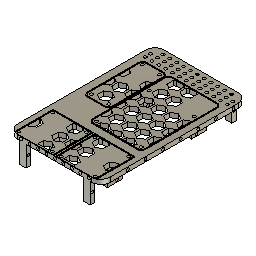
goose chassis v5 (Autodesk Fusion 360 design; units mm, degrees)
Autodesk Fusion 360 part; units mm, degrees
(part 1 of 2)
sketch "Sketch1" plane through (0, 0, 0) normal (0, 0, 1) x (1, 0, 0)
  line L0 (0, 0) -> (60, 0)
  line L1 (60, 0) -> (60, 100)
  line L2 (60, 100) -> (0, 100)
  line L3 (0, 100) -> (0, 0)
  line L4 (2, 92.9) -> (58, 92.9) construction
  line L5 (58, 92.9) -> (58, 7.1) construction
  line L6 (58, 7.1) -> (2, 7.1) construction
  line L7 (2, 7.1) -> (2, 92.9) construction
  line L8 (30, 92.9) -> (30, 7.1) construction
  line L9 (58, 50) -> (2, 50) construction
  line L10 (30, 100) -> (30, 0) construction
  line L11 (0, 50) -> (60, 50) construction
  line L12 (5.5, 89.5721) -> (54.5, 89.5721) construction
  line L13 (54.5, 89.5721) -> (54.5, 31.5721) construction
  line L14 (54.5, 31.5721) -> (5.5, 31.5721) construction
  line L15 (5.5, 31.5721) -> (5.5, 89.5721) construction
  line L16 (30, 89.5721) -> (30, 31.5721) construction
  circle A0 centre (5.5, 89.5721) radius 1.6
  circle A1 centre (54.5, 89.5721) radius 1.6
  circle A2 centre (54.5, 31.5721) radius 1.6
  circle A3 centre (5.5, 31.5721) radius 1.6
  line L17 (0, 100) -> (0, 140)
  line L18 (60, 100) -> (60, 140)
  line L19 (0, 140) -> (60, 140)
  dimension "d1" = 60
  dimension "d2" = 100
  dimension "d3" = 56
  dimension "d4" = 85.8
  dimension "d5" = 49
  dimension "d6" = 58
  dimension "d7" = 3.2
  dimension "d8" = 3.2
  dimension "d9" = 3.2
  dimension "d10" = 3.2
  dimension "d11" = 40
  dimension "d12" = 40
  constraint horizontal L0
  constraint vertical L1
  constraint horizontal L2
  constraint vertical L3
  constraint coincident L0.start L3.end
  constraint horizontal L4
  constraint vertical L5
  constraint horizontal L6
  constraint vertical L7
  constraint midpoint L4 L8.start
  constraint midpoint L6 L8.end
  constraint midpoint L5 L9.start
  constraint midpoint L7 L9.end
  constraint midpoint L2 L10.start
  constraint midpoint L0 L10.end
  constraint midpoint L3 L11.start
  constraint midpoint L1 L11.end
  constraint collinear L9 L11
  constraint collinear L8 L10
  constraint horizontal L12
  constraint vertical L13
  constraint horizontal L14
  constraint vertical L15
  constraint midpoint L12 L16.start
  constraint midpoint L14 L16.end
  constraint collinear L10 L16
  constraint coincident L12.start L15.end
  constraint coincident L12.end L13.start
  constraint coincident L13.end L14.start
  constraint coincident L14.end L15.start
  constraint perpendicular L2 L17
  constraint perpendicular L2 L18
  measures "d1" distance of L0.start L0.end
  measures "d2" distance of L0.start L2.end
  measures "d3" distance of L4.start L4.end
  measures "d4" distance of L4.start L6.end
  measures "d5" distance of L12.start L12.end
  measures "d6" distance of L12.start L14.end
  measures "d7" diameter of A0
  measures "d8" diameter of A1
  measures "d9" diameter of A2
  measures "d10" diameter of A3
  measures "d11" distance of L2.end L17.end
  measures "d12" distance of L1.end L18.end
extrude "Extrude1" add sketch "Sketch1" along normal blind 5 contours L0 L1 L2 L3 | L2 L17 L18 L19 | A0 | A1 | A2 | A3 makes body 1
sketch "Sketch2" plane through (0, 0, 0) normal (0, 0, 1) x (1, 0, 0)
  line L0 (0, 0) -> (19, 0) construction
  line L1 (19, 0) -> (19, 70) construction
  line L2 (19, 70) -> (0, 70) construction
  line L3 (0, 70) -> (0, 0) construction
  line L4 (9.5, 70) -> (9.5, 0) construction
  line L5 (19, 35) -> (0, 35) construction
  line L6 (19, 0) -> (12, 0)
  line L7 (12, 0) -> (12, 5)
  line L8 (12, 5) -> (19, 5)
  line L9 (19, 5) -> (19, 0)
  line L10 (19, 26) -> (29, 26)
  line L11 (29, 26) -> (29, 42)
  line L12 (29, 42) -> (19, 42)
  line L13 (19, 42) -> (19, 26)
  line L14 (0, 0) -> (60, 0) construction
  line L15 (60, 0) -> (60, 140) construction
  line L16 (60, 140) -> (0, 140) construction
  line L17 (0, 140) -> (0, 0) construction
  line L18 (30, 140) -> (30, 0) construction
  line L19 (60, 70) -> (0, 70) construction
  line L20 (41, 26) -> (31, 26)
  line L21 (31, 26) -> (31, 42)
  line L22 (41, 42) -> (41, 26)
  line L23 (31, 42) -> (41, 42)
  line L24 (41, 0) -> (48, 0)
  line L25 (48, 0) -> (48, 5)
  line L26 (41, 5) -> (41, 0)
  line L27 (48, 5) -> (41, 5)
  line L28 (41, 114) -> (31, 114)
  line L29 (31, 114) -> (31, 98)
  line L30 (41, 98) -> (41, 114)
  line L31 (31, 98) -> (41, 98)
  line L32 (19, 114) -> (29, 114)
  line L33 (29, 114) -> (29, 98)
  line L34 (19, 98) -> (19, 114)
  line L35 (29, 98) -> (19, 98)
  line L36 (19, 140) -> (12, 140)
  line L37 (12, 140) -> (12, 135)
  line L38 (19, 135) -> (19, 140)
  line L39 (12, 135) -> (19, 135)
  line L40 (41, 140) -> (48, 140)
  line L41 (48, 140) -> (48, 135)
  line L42 (41, 135) -> (41, 140)
  line L43 (48, 135) -> (41, 135)
  dimension "d15" = 19
  dimension "d16" = 70
  dimension "d17" = 7
  dimension "d18" = 5
  dimension "d19" = 12
  dimension "d20" = 10
  dimension "d21" = 16
  dimension "d22" = 42
  constraint horizontal L0
  constraint vertical L1
  constraint horizontal L2
  constraint vertical L3
  constraint coincident L0.start L3.end
  constraint midpoint L2 L4.start
  constraint midpoint L0 L4.end
  constraint midpoint L1 L5.start
  constraint midpoint L3 L5.end
  constraint horizontal L6
  constraint vertical L7
  constraint horizontal L8
  constraint vertical L9
  constraint coincident L0 L1.start
  constraint horizontal L10
  constraint vertical L11
  constraint horizontal L12
  constraint vertical L13
  constraint coincident L1 L10.start
  constraint horizontal L14
  constraint vertical L15
  constraint horizontal L16
  constraint vertical L17
  constraint midpoint L16 L18.start
  constraint midpoint L14 L18.end
  constraint midpoint L15 L19.start
  constraint perpendicular L3 L19
  constraint symmetric L0.end L18 L24.start
  constraint symmetric L6.end L18 L24.end
  constraint symmetric L7.end L18 L25.end
  constraint symmetric L8.end L18 L26.start
  constraint symmetric L10.start L18 L20.start
  constraint symmetric L10.end L18 L20.end
  constraint symmetric L11.end L18 L21.end
  constraint symmetric L12.end L18 L22.start
  constraint symmetric L0.end L19 L36.start
  constraint symmetric L6.end L19 L36.end
  constraint symmetric L7.end L19 L37.end
  constraint symmetric L8.end L19 L38.start
  constraint symmetric L10.start L19 L32.start
  constraint symmetric L10.end L19 L32.end
  constraint symmetric L11.end L19 L33.end
  constraint symmetric L12.end L19 L34.start
  constraint symmetric L19 L20.start L28.start
  constraint symmetric L19 L20.end L28.end
  constraint symmetric L19 L21.end L29.end
  constraint symmetric L19 L22.start L30.start
  constraint symmetric L19 L24.start L40.start
  constraint symmetric L19 L24.end L40.end
  constraint symmetric L19 L25.end L41.end
  constraint symmetric L19 L26.start L42.start
  measures "d15" distance of L0.start L0.end
  measures "d16" distance of L0.start L2.end
  measures "d17" distance of L0.end L6.end
  measures "d18" distance of L0.end L8.end
  measures "d19" distance of L3 L7
  measures "d20" distance of L10.start L10.end
  measures "d21" distance of L10.start L12.end
  measures "d22" distance of L12 L14
extrude "Extrude2" add sketch "Sketch2" against normal blind 22.5 bodies 1
sketch "Sketch3" plane through (12, 0, 0) normal (-1, 0, 0) x (0, -1, 0)
  line L0 (0, 0) -> (-5, 0)
  line L1 (-5, 0) -> (-5, -22.5)
  line L2 (-5, -22.5) -> (0, -22.5)
  line L3 (0, -22.5) -> (0, 0)
  line L4 (-2.5, 0) -> (-2.5, -11.5) construction
  circle A0 centre (-2.5, -11.5) radius 1.6
  circle A1 centre (-36.5, -2.5) radius 1.6
  circle A2 centre (-36.5, -20) radius 1.6
  line L5 (-140, 0) -> (0, 0)
  line L6 (-42, 0) -> (-42, -22.5)
  dimension "d25" = 11.5
  dimension "d26" = 3.2
  dimension "d27" = 3.2
  dimension "d28" = 3.2
  dimension "d29" = 2.5
  dimension "d30" = 5.5
  dimension "d31" = 20
  dimension "d32" = 5.5
  constraint midpoint L0 L4.start
  constraint perpendicular L0 L4
  constraint coincident L4.end A0.centre
  measures "d25" distance of L4.start L4.end
  measures "d26" diameter of A0
  measures "d27" diameter of A1
  measures "d28" diameter of A2
  measures "d29" distance of A1.centre L5
  measures "d30" distance of A1.centre L6
  measures "d31" distance of A2.centre L5
  measures "d32" distance of A2.centre L6
extrude "Extrude3" cut sketch "Sketch3" against normal blind 40 contours A0 | A1 | A2 bodies 1
ref_plane "WorkPlane1" through (30, 70, -8.75) normal (0, -1, 0) x (1, 0, 0)
mirror "Mirror1" about plane through (30, 70, -8.75) normal (0, -1, 0) of "Extrude3"
copy_body "Body->Comp1" bodies 1 removing the originals makes body 2 in component "chassis"
ref_plane "WorkPlane1" through (30, 80, -8.75) normal (0, -1, 0) x (1, 0, 0) in component "chassis"
split "Split1" by plane through (30, 80, -8.75) normal (0, -1, 0) bodies 2 makes body 3 at (20, 53.3333, 5) in component "chassis"
move_body "Move1" bodies 2 to x (1, 0, 0) y (0, 1, 0) z (0, 0, 1) at (0, 20, 0) in component "chassis"
loft "Loft1" add section 1 face at (20, 80, 1.6667) section 2 face at (20, 100, 1.6667) on bodies 2 3 bodies 2 3 in component "chassis"
ref_plane "WorkPlane2" through (30, 80, 2.5) normal (-1, 0, 0) x (0, -1, 0) in component "chassis"
split "Split2" by plane through (30, 80, 2.5) normal (-1, 0, 0) bodies 2 makes body 4 at (10, 106.6667, 5) in component "chassis"
move_body "Move2" bodies 2 to x (1, 0, 0) y (0, 1, 0) z (0, 0, 1) at (41, 0, 0) in component "chassis"
loft "Loft2" add section 1 face at (30, 53.3333, 3.3333) section 2 face at (71, 53.3333, 3.3333) on bodies 2 4 bodies 2 4 in component "chassis"
sketch "Sketch6" plane through (0, 0, 5) normal (0, 0, 1) x (-1, 0, 0)
  line L0 (-101, -160) -> (0, -160)
  line L1 (0, -160) -> (0, 0)
  line L2 (0, 0) -> (-101, 0)
  line L3 (-101, 0) -> (-101, -160)
  line L4 (-89.5, -55.4279) -> (-40.5, -55.4279) construction
  line L5 (-40.5, -55.4279) -> (-40.5, -113.4279) construction
  line L6 (-40.5, -113.4279) -> (-89.5, -113.4279) construction
  line L7 (-89.5, -113.4279) -> (-89.5, -55.4279) construction
  line L8 (-93, -52.1) -> (-37, -52.1) construction
  line L9 (-37, -52.1) -> (-37, -137.9) construction
  line L10 (-93, -137.9) -> (-93, -52.1) construction
  line L11 (-37, -137.9) -> (-93, -137.9) construction
  circle A0 centre (-40.5, -113.4279) radius 1.6
  circle A1 centre (-89.5, -113.4279) radius 1.6
  circle A2 centre (-40.5, -55.4279) radius 1.6
  circle A3 centre (-89.5, -55.4279) radius 1.6
  circle A4 centre (-54.9377, -39.4681) radius 1.6
  circle A5 centre (-54.9377, -2.6181) radius 1.6
  line L12 (0, -80) -> (-101, -80) construction
  line L13 (-31.1163, -133.9449) -> (-31.1163, -78.4449) construction
  line L14 (-31.1163, -78.4449) -> (-12.1163, -78.4449) construction
  line L15 (-12.1163, -78.4449) -> (-12.1163, -133.9449) construction
  line L16 (-12.1163, -133.9449) -> (-31.1163, -133.9449) construction
  line L17 (-34.8217, -137.6274) -> (-34.8217, -74.6274) construction
  line L18 (-34.8217, -74.6274) -> (-8.8217, -74.6274) construction
  line L19 (-8.8217, -74.6274) -> (-8.8217, -137.6274) construction
  line L20 (-8.8217, -137.6274) -> (-34.8217, -137.6274) construction
  circle A6 centre (-31.1163, -133.9449) radius 1.6
  circle A7 centre (-31.1163, -78.4449) radius 1.6
  circle A8 centre (-12.1163, -78.4449) radius 1.6
  circle A9 centre (-12.1163, -133.9449) radius 1.6
  circle A10 centre (-91.9377, -2.6181) radius 1.6
  circle A11 centre (-91.9377, -39.4681) radius 1.6
  line L21 (-101, 0) -> (0, 0) construction
  line L22 (0, 0) -> (0, -160) construction
  line L23 (0, -160) -> (-101, -160) construction
  line L24 (-101, -160) -> (-101, 0) construction
  line L25 (-50, 0) -> (-50.5, -160) construction
  circle A12 centre (-8.0795, -2.8802) radius 1.6
  circle A13 centre (-8.3098, -39.7295) radius 1.6
  circle A14 centre (-45.3091, -39.4982) radius 1.6
  circle A15 centre (-45.0788, -2.6489) radius 1.6
  dimension "d77" = 56
  dimension "d78" = 85.8
  dimension "d79" = 49
  dimension "d80" = 58
  dimension "d81" = 3.2
  dimension "d82" = 3.2
  dimension "d83" = 3.2
  dimension "d84" = 3.2
  dimension "d85" = 55.5
  dimension "d86" = 19
  dimension "d87" = 63
  dimension "d88" = 26
  dimension "d89" = 3.2
  dimension "d90" = 3.2
  dimension "d91" = 3.2
  dimension "d92" = 3.2
  constraint horizontal L8
  constraint vertical L9
  constraint horizontal L11
  constraint vertical L10
  constraint horizontal L4
  constraint vertical L5
  constraint horizontal L6
  constraint vertical L7
  constraint coincident L4.start L7.end
  constraint coincident L4.end L5.start
  constraint coincident L5.end L6.start
  constraint coincident L6.end L7.start
  constraint midpoint L1 L12.start
  constraint midpoint L3 L12.end
  constraint coincident L13.start L16.end
  constraint coincident L13.end L14.start
  constraint coincident L14.end L15.start
  constraint coincident L15.end L16.start
  constraint horizontal L21
  constraint vertical L22
  constraint horizontal L23
  constraint vertical L24
  constraint coincident L0.end L1.start
  constraint coincident L2.end L3.start
  constraint coincident L21 L25.start
  constraint midpoint L23 L25.end
  constraint symmetric A4 L25 A14
  constraint symmetric A5 L25 A15
  constraint symmetric A10 L25 A12
  constraint symmetric A11 L25 A13
  measures "d77" distance of L8.start L8.end
  measures "d78" distance of L8.start L10.start
  measures "d79" distance of L4.start L4.end
  measures "d80" distance of L6.end L4.start
  measures "d81" diameter of A3
  measures "d82" diameter of A2
  measures "d83" diameter of A0
  measures "d84" diameter of A1
  measures "d85" distance of L13.start L13.end
  measures "d86" distance of L13.start L15.end
  measures "d87" distance of L17.start L17.end
  measures "d88" distance of L17.start L19.end
  measures "d89" diameter of A6
  measures "d90" diameter of A7
  measures "d91" diameter of A8
  measures "d92" diameter of A9
extrude "Extrude1'" add sketch "Sketch6" against normal blind 5 contours A0 | A1 | A2 | A3 | A4 | A5 | A6 | A7 | A8 | A9 | A10 | A11 | A12 | A13 | A14 | A15 bodies 2 in component "chassis"
extrude "Extrude2'" cut sketch "Sketch6" against normal blind 5 contours A0 | A1 | A2 | A3 | A4 | A5 | A6 | A7 | A8 | A9 | A10 | A11 | A12 | A13 | A14 | A15 bodies 2 in component "chassis"
fillet "Fillet3" radius 10 4 edges at (101, 0, 2.5) (0, 0, 2.5) (0, 160, 2.5) (101, 160, 2.5) on bodies 2 in component "chassis"
sketch "Sketch7" plane through (0, 0, 5) normal (0, 0, 1) x (-1, 0, 0)
  circle A0 centre (-45.3091, -39.4982) radius 1.6
  circle A1 centre (-54.9377, -2.6181) radius 1.6
  circle A2 centre (-40.5, -55.4279) radius 1.6
  circle A3 centre (-89.5, -55.4279) radius 1.6
  circle A4 centre (-31.1163, -133.9449) radius 1.6
  circle A5 centre (-40.5, -113.4279) radius 1.6
  circle A6 centre (-8.3098, -39.7295) radius 1.6
  circle A7 centre (-91.9377, -39.4681) radius 1.6
  circle A8 centre (-45.0788, -2.6489) radius 1.6
  circle A9 centre (-12.1163, -78.4449) radius 1.6
  circle A10 centre (-31.1163, -78.4449) radius 1.6
  circle A11 centre (-54.9377, -39.4681) radius 1.6
  circle A12 centre (-12.1163, -133.9449) radius 1.6
  circle A13 centre (-89.5, -113.4279) radius 1.6
  circle A14 centre (-8.0795, -2.8802) radius 1.6
  circle A15 centre (-91.9377, -2.6181) radius 1.6
  arc A16 (-101, -150) -> (-91, -160) centre (-91, -150) ccw
  line L0 (-91, -160) -> (-10, -160)
  arc A17 (-10, -160) -> (0, -150) centre (-10, -150) ccw
  line L1 (0, -150) -> (0, -10)
  arc A18 (0, -10) -> (-10, 0) centre (-10, -10) ccw
  line L2 (-10, 0) -> (-91, 0)
  arc A19 (-91, 0) -> (-101, -10) centre (-91, -10) ccw
  line L3 (-101, -10) -> (-101, -150)
  line L4 (-91.9377, -2.6181) -> (-54.9377, -2.6181) construction
  line L5 (-54.9377, -2.6181) -> (-54.9377, -39.4681) construction
  line L6 (-54.9377, -39.4681) -> (-91.9377, -39.4681) construction
  line L7 (-91.9377, -39.4681) -> (-91.9377, -2.6181) construction
  line L8 (-94.4377, -41.9681) -> (-94.4377, -0.1181)
  line L9 (-94.4377, -0.1181) -> (-52.4377, -0.1181)
  line L10 (-52.4377, -0.1181) -> (-52.4377, -41.9681)
  line L11 (-52.4377, -41.9681) -> (-94.4377, -41.9681)
  line L12 (-41, -137.9) -> (-89, -137.9)
  line L13 (-93, -133.9) -> (-93, -56.1)
  line L14 (-89, -52.1) -> (-41, -52.1)
  line L15 (-37, -56.1) -> (-37, -133.9)
  line L16 (-12.8217, -137.6274) -> (-30.8217, -137.6274)
  line L17 (-34.8217, -133.6274) -> (-34.8217, -78.6274)
  line L18 (-30.8217, -74.6274) -> (-12.8217, -74.6274)
  line L19 (-8.8217, -78.6274) -> (-8.8217, -133.6274)
  arc A20 (-89, -52.1) -> (-93, -56.1) centre (-89, -56.1) ccw
  arc A21 (-37, -56.1) -> (-41, -52.1) centre (-41, -56.1) ccw
  arc A22 (-41, -137.9) -> (-37, -133.9) centre (-41, -133.9) ccw
  arc A23 (-93, -133.9) -> (-89, -137.9) centre (-89, -133.9) ccw
  arc A24 (-34.8217, -133.6274) -> (-30.8217, -137.6274) centre (-30.8217, -133.6274) ccw
  arc A25 (-12.8217, -137.6274) -> (-8.8217, -133.6274) centre (-12.8217, -133.6274) ccw
  arc A26 (-8.8217, -78.6274) -> (-12.8217, -74.6274) centre (-12.8217, -78.6274) ccw
  arc A27 (-30.8217, -74.6274) -> (-34.8217, -78.6274) centre (-30.8217, -78.6274) ccw
  line L20 (-50.5, 0) -> (-50.5, -160) construction
  line L21 (-6.5623, -41.9681) -> (-6.5623, -0.1181)
  line L22 (-6.5623, -0.1181) -> (-48.5623, -0.1181)
  line L23 (-48.5623, -0.1181) -> (-48.5623, -41.9681)
  line L24 (-48.5623, -41.9681) -> (-6.5623, -41.9681)
  line L25 (-95.4377, 0.8819) -> (-51.4377, 0.8819)
  line L26 (-51.4377, 0.8819) -> (-51.4377, -42.9681)
  line L27 (-51.4377, -42.9681) -> (-95.4377, -42.9681)
  line L28 (-95.4377, -42.9681) -> (-95.4377, 0.8819)
  line L29 (-5.5623, 0.8819) -> (-49.5623, 0.8819)
  line L30 (-49.5623, 0.8819) -> (-49.5623, -42.9681)
  line L31 (-49.5623, -42.9681) -> (-5.5623, -42.9681)
  line L32 (-5.5623, -42.9681) -> (-5.5623, 0.8819)
  arc A28 (-36, -56.1) -> (-41, -51.1) centre (-41, -56.1) ccw
  line L33 (-89, -51.1) -> (-41, -51.1)
  arc A29 (-89, -51.1) -> (-94, -56.1) centre (-89, -56.1) ccw
  line L34 (-94, -133.9) -> (-94, -56.1)
  arc A30 (-94, -133.9) -> (-89, -138.9) centre (-89, -133.9) ccw
  line L35 (-41, -138.9) -> (-89, -138.9)
  arc A31 (-41, -138.9) -> (-36, -133.9) centre (-41, -133.9) ccw
  line L36 (-36, -56.1) -> (-36, -133.9)
  arc A32 (-7.8217, -78.6274) -> (-12.8217, -73.6274) centre (-12.8217, -78.6274) ccw
  line L37 (-30.8217, -73.6274) -> (-12.8217, -73.6274)
  arc A33 (-30.8217, -73.6274) -> (-35.8217, -78.6274) centre (-30.8217, -78.6274) ccw
  line L38 (-35.8217, -133.6274) -> (-35.8217, -78.6274)
  arc A34 (-35.8217, -133.6274) -> (-30.8217, -138.6274) centre (-30.8217, -133.6274) ccw
  line L39 (-12.8217, -138.6274) -> (-30.8217, -138.6274)
  arc A35 (-12.8217, -138.6274) -> (-7.8217, -133.6274) centre (-12.8217, -133.6274) ccw
  line L40 (-7.8217, -78.6274) -> (-7.8217, -133.6274)
  point P0 (-93.0412, -137.3397)
  point P1 (-93.0412, -51.5397)
  point P2 (-37.0412, -51.5397)
  point P3 (-34.8217, -127.6274)
  point P4 (-8.8217, -127.6274)
  point P5 (-93, -137.9)
  point P6 (-93, -52.1)
  point P7 (-37, -52.1)
  point P8 (-34.8217, -137.6274)
  point P9 (-34.8217, -74.6274)
  point P10 (-8.8217, -137.6274)
  dimension "d112" = -2.5
  dimension "d113" = 56
  dimension "d114" = 85.8
  dimension "d115" = 63
  dimension "d116" = 26
  dimension "d117" = 4
  dimension "d118" = -1
  dimension "d119" = 1
  dimension "d120" = -1
  dimension "d121" = -1
  constraint horizontal L4
  constraint vertical L5
  constraint horizontal L6
  constraint vertical L7
  constraint coincident A11.centre L5.end
  constraint coincident A15.centre L4.start
  constraint horizontal L14
  constraint vertical L15
  constraint horizontal L12
  constraint vertical L13
  constraint coincident P6 L13
  constraint coincident P6 L14
  constraint tangent L13 A20
  constraint tangent L14 A20
  constraint coincident P7 L14
  constraint coincident P7 L15
  constraint tangent L14 A21
  constraint tangent L15 A21
  constraint equal A20 A21
  constraint tangent L12 A22
  constraint tangent L15 A22
  constraint equal A20 A22
  constraint coincident P5 L12
  constraint coincident P5 L13
  constraint tangent L12 A23
  constraint tangent L13 A23
  constraint equal A20 A23
  constraint coincident P8 L16
  constraint coincident P8 L17
  constraint tangent L16 A24
  constraint tangent L17 A24
  constraint equal A20 A24
  constraint coincident P10 L16
  constraint coincident P10 L19
  constraint tangent L16 A25
  constraint tangent L19 A25
  constraint equal A20 A25
  constraint tangent L18 A26
  constraint tangent L19 A26
  constraint equal A20 A26
  constraint coincident P9 L17
  constraint coincident P9 L18
  constraint tangent L17 A27
  constraint tangent L18 A27
  constraint equal A20 A27
  constraint midpoint L2 L20.start
  constraint midpoint L0 L20.end
  constraint symmetric L8.start L20 L21.start
  constraint symmetric L8.end L20 L21.end
  constraint symmetric L9.end L20 L22.end
  constraint symmetric L10.end L20 L23.end
  measures "d113" distance of P6 P7
  measures "d114" distance of P5 P6
  measures "d115" distance of P8 P9
  measures "d116" distance of P8 P10
  measures "d117" radius of A20
extrude "Extrude3'" cut sketch "Sketch7" against normal blind 0.5 contours A14 A18 L2 L21 L22 L23 L24 L30 L31 L32 | L2 A19 L8 L9 L10 L11 L26 L27 L28 | A28 L33 A29 L34 A30 L35 A31 L36 | A32 L37 A33 L38 A34 L39 A35 L40 bodies 2 in component "chassis"
sketch "Sketch8" plane through (0, 0, 5) normal (0, 0, 1) x (-1, 0, 0)
  line L0 (-95.4377, -42.9681) -> (-95.4377, -1.0386)
  arc A0 (-95.4377, -1.0386) -> (-101, -10) centre (-91, -10) ccw
  line L1 (-101, -10) -> (-101, -150)
  arc A1 (-101, -150) -> (-91, -160) centre (-91, -150) ccw
  line L2 (-91, -160) -> (-10, -160)
  arc A2 (-10, -160) -> (0, -150) centre (-10, -150) ccw
  line L3 (0, -150) -> (0, -10)
  arc A3 (0, -10) -> (-5.5623, -1.0386) centre (-10, -10) ccw
  line L4 (-5.5623, -1.0386) -> (-5.5623, -42.9681)
  line L5 (-5.5623, -42.9681) -> (-49.5623, -42.9681)
  line L6 (-49.5623, -42.9681) -> (-49.5623, 0)
  line L7 (-49.5623, 0) -> (-51.4377, 0)
  line L8 (-51.4377, 0) -> (-51.4377, -42.9681)
  line L9 (-51.4377, -42.9681) -> (-95.4377, -42.9681)
  line L10 (-94, -133.9) -> (-94, -56.1)
  arc A4 (-89, -51.1) -> (-94, -56.1) centre (-89, -56.1) ccw
  line L11 (-89, -51.1) -> (-41, -51.1)
  arc A5 (-36, -56.1) -> (-41, -51.1) centre (-41, -56.1) ccw
  line L12 (-36, -56.1) -> (-36, -133.9)
  arc A6 (-41, -138.9) -> (-36, -133.9) centre (-41, -133.9) ccw
  line L13 (-41, -138.9) -> (-89, -138.9)
  arc A7 (-94, -133.9) -> (-89, -138.9) centre (-89, -133.9) ccw
  line L14 (-35.8217, -133.6274) -> (-35.8217, -78.6274)
  arc A8 (-30.8217, -73.6274) -> (-35.8217, -78.6274) centre (-30.8217, -78.6274) ccw
  line L15 (-30.8217, -73.6274) -> (-12.8217, -73.6274)
  arc A9 (-7.8217, -78.6274) -> (-12.8217, -73.6274) centre (-12.8217, -78.6274) ccw
  line L16 (-7.8217, -78.6274) -> (-7.8217, -133.6274)
  arc A10 (-12.8217, -138.6274) -> (-7.8217, -133.6274) centre (-12.8217, -133.6274) ccw
  line L17 (-12.8217, -138.6274) -> (-30.8217, -138.6274)
  arc A11 (-35.8217, -133.6274) -> (-30.8217, -138.6274) centre (-30.8217, -133.6274) ccw
  line L18 (-65, -51.1) -> (-65, -138.9) construction
  line L19 (-36, -95) -> (-94, -95) construction
  line L20 (-21.8217, -73.6274) -> (-21.8217, -138.6274) construction
  line L21 (-35.8217, -106.1274) -> (-7.8217, -106.1274) construction
  line L22 (-95.4377, -22.0034) -> (-51.4377, -21.4841) construction
  line L23 (-73.4377, -42.9681) -> (-73.4377, 0) construction
  line L24 (-94.007, -10.6431) -> (-92.5355, -11.4927)
  line L25 (-92.5355, -11.4927) -> (-86.5355, -8.0286)
  line L26 (-86.5355, -8.0286) -> (-86.5355, -2.0505)
  line L27 (-84.3689, -2.0505) -> (-84.3689, -8.0286)
  line L28 (-84.3689, -8.0286) -> (-78.3689, -11.4927)
  line L29 (-78.3689, -11.4927) -> (-72.3689, -8.0286)
  line L30 (-72.3689, -8.0286) -> (-72.3689, -2.0505)
  line L31 (-70.2022, -2.0505) -> (-70.2022, -8.0286)
  line L32 (-70.2022, -8.0286) -> (-64.2022, -11.4927)
  line L33 (-64.2022, -11.4927) -> (-58.2022, -8.0286)
  line L34 (-58.2022, -8.0286) -> (-58.2022, -2.0505)
  line L35 (-41.8689, -2.0505) -> (-41.8689, -8.0286)
  line L36 (-41.8689, -8.0286) -> (-35.8689, -11.4927)
  line L37 (-35.8689, -11.4927) -> (-29.8689, -8.0286)
  line L38 (-29.8689, -8.0286) -> (-29.8689, -2.0505)
  line L39 (-27.7022, -2.0505) -> (-27.7022, -8.0286)
  line L40 (-27.7022, -8.0286) -> (-21.7022, -11.4927)
  line L41 (-21.7022, -11.4927) -> (-15.7022, -8.0286)
  line L42 (-15.7022, -8.0286) -> (-15.7022, -2.0505)
  line L43 (-13.5355, -2.0505) -> (-13.5355, -8.0286)
  line L44 (-13.5355, -8.0286) -> (-7.5355, -11.4927)
  line L45 (-7.5355, -11.4927) -> (-7, -11.1835)
  line L46 (-94.007, -26.6431) -> (-92.5355, -27.4927)
  line L47 (-92.5355, -27.4927) -> (-86.5355, -24.0286)
  line L48 (-86.5355, -24.0286) -> (-86.5355, -17.1004)
  line L49 (-92.5355, -13.6363) -> (-94.007, -14.4858)
  line L50 (-86.5355, -17.1004) -> (-92.5355, -13.6363)
  line L51 (-84.3689, -17.1004) -> (-84.3689, -24.0286)
  line L52 (-84.3689, -24.0286) -> (-78.3689, -27.4927)
  line L53 (-78.3689, -27.4927) -> (-72.3689, -24.0286)
  line L54 (-72.3689, -24.0286) -> (-72.3689, -17.1004)
  line L55 (-78.3689, -13.6363) -> (-84.3689, -17.1004)
  line L56 (-72.3689, -17.1004) -> (-78.3689, -13.6363)
  line L57 (-70.2022, -17.1004) -> (-70.2022, -24.0286)
  line L58 (-70.2022, -24.0286) -> (-64.2022, -27.4927)
  line L59 (-64.2022, -27.4927) -> (-58.2022, -24.0286)
  line L60 (-58.2022, -24.0286) -> (-58.2022, -17.1004)
  line L61 (-64.2022, -13.6363) -> (-70.2022, -17.1004)
  line L62 (-58.2022, -17.1004) -> (-64.2022, -13.6363)
  line L63 (-56.0355, -17.1004) -> (-56.0355, -24.0286)
  line L64 (-44.0355, -24.0286) -> (-44.0355, -17.1004)
  line L65 (-44.0355, -17.1004) -> (-47.9856, -14.8198)
  line L66 (-41.8689, -17.1004) -> (-41.8689, -24.0286)
  line L67 (-41.8689, -24.0286) -> (-35.8689, -27.4927)
  line L68 (-35.8689, -27.4927) -> (-29.8689, -24.0286)
  line L69 (-29.8689, -24.0286) -> (-29.8689, -17.1004)
  line L70 (-35.8689, -13.6363) -> (-41.8689, -17.1004)
  line L71 (-29.8689, -17.1004) -> (-35.8689, -13.6363)
  line L72 (-27.7022, -17.1004) -> (-27.7022, -24.0286)
  line L73 (-27.7022, -24.0286) -> (-21.7022, -27.4927)
  line L74 (-21.7022, -27.4927) -> (-15.7022, -24.0286)
  line L75 (-15.7022, -24.0286) -> (-15.7022, -17.1004)
  line L76 (-21.7022, -13.6363) -> (-27.7022, -17.1004)
  line L77 (-15.7022, -17.1004) -> (-21.7022, -13.6363)
  line L78 (-13.5355, -17.1004) -> (-13.5355, -24.0286)
  line L79 (-13.5355, -24.0286) -> (-7.5355, -27.4927)
  line L80 (-7.5355, -13.6363) -> (-13.5355, -17.1004)
  line L81 (-7, -13.9455) -> (-7.5355, -13.6363)
  line L82 (-84.3689, -33.1004) -> (-84.3689, -40.0286)
  line L83 (-72.3689, -40.0286) -> (-72.3689, -33.1004)
  line L84 (-78.3689, -29.6363) -> (-84.3689, -33.1004)
  line L85 (-72.3689, -33.1004) -> (-78.3689, -29.6363)
  line L86 (-70.2022, -33.1004) -> (-70.2022, -40.0286)
  line L87 (-60.7508, -41.5) -> (-58.2022, -40.0286)
  line L88 (-58.2022, -40.0286) -> (-58.2022, -33.1004)
  line L89 (-64.2022, -29.6363) -> (-70.2022, -33.1004)
  line L90 (-58.2022, -33.1004) -> (-64.2022, -29.6363)
  line L91 (-41.8689, -33.1004) -> (-41.8689, -40.0286)
  line L92 (-29.8689, -40.0286) -> (-29.8689, -33.1004)
  line L93 (-35.8689, -29.6363) -> (-41.8689, -33.1004)
  line L94 (-29.8689, -33.1004) -> (-35.8689, -29.6363)
  line L95 (-27.7022, -33.1004) -> (-27.7022, -40.0286)
  line L96 (-15.7022, -40.0286) -> (-15.7022, -33.1004)
  line L97 (-21.7022, -29.6363) -> (-27.7022, -33.1004)
  line L98 (-15.7022, -33.1004) -> (-21.7022, -29.6363)
  line L99 (-84.3689, -52.5645) -> (-84.3689, -56.0286)
  line L100 (-84.3689, -56.0286) -> (-78.3689, -59.4927)
  line L101 (-78.3689, -59.4927) -> (-72.3689, -56.0286)
  line L102 (-72.3689, -56.0286) -> (-72.3689, -52.5645)
  line L103 (-70.2022, -52.5645) -> (-70.2022, -56.0286)
  line L104 (-70.2022, -56.0286) -> (-64.2022, -59.4927)
  line L105 (-64.2022, -59.4927) -> (-58.2022, -56.0286)
  line L106 (-58.2022, -56.0286) -> (-58.2022, -52.5645)
  line L107 (-56.0355, -52.5645) -> (-56.0355, -56.0286)
  line L108 (-56.0355, -56.0286) -> (-50.0355, -59.4927)
  line L109 (-50.0355, -59.4927) -> (-44.0355, -56.0286)
  line L110 (-44.0355, -56.0286) -> (-44.0355, -52.5645)
  line L111 (-92.5355, -75.4927) -> (-86.5355, -72.0286)
  line L112 (-86.5355, -72.0286) -> (-86.5355, -65.1004)
  line L113 (-86.5355, -65.1004) -> (-92.5355, -61.6363)
  line L114 (-84.3689, -65.1004) -> (-84.3689, -72.0286)
  line L115 (-84.3689, -72.0286) -> (-78.3689, -75.4927)
  line L116 (-78.3689, -75.4927) -> (-72.3689, -72.0286)
  line L117 (-72.3689, -72.0286) -> (-72.3689, -65.1004)
  line L118 (-78.3689, -61.6363) -> (-84.3689, -65.1004)
  line L119 (-72.3689, -65.1004) -> (-78.3689, -61.6363)
  line L120 (-70.2022, -65.1004) -> (-70.2022, -72.0286)
  line L121 (-70.2022, -72.0286) -> (-64.2022, -75.4927)
  line L122 (-64.2022, -75.4927) -> (-58.2022, -72.0286)
  line L123 (-58.2022, -72.0286) -> (-58.2022, -65.1004)
  line L124 (-64.2022, -61.6363) -> (-70.2022, -65.1004)
  line L125 (-58.2022, -65.1004) -> (-64.2022, -61.6363)
  line L126 (-56.0355, -65.1004) -> (-56.0355, -72.0286)
  line L127 (-56.0355, -72.0286) -> (-50.0355, -75.4927)
  line L128 (-50.0355, -75.4927) -> (-44.0355, -72.0286)
  line L129 (-44.0355, -72.0286) -> (-44.0355, -65.1004)
  line L130 (-50.0355, -61.6363) -> (-56.0355, -65.1004)
  line L131 (-44.0355, -65.1004) -> (-50.0355, -61.6363)
  line L132 (-41.8689, -65.1004) -> (-41.8689, -72.0286)
  line L133 (-92.5355, -91.4927) -> (-86.5355, -88.0286)
  line L134 (-86.5355, -88.0286) -> (-86.5355, -81.1004)
  line L135 (-86.5355, -81.1004) -> (-92.5355, -77.6363)
  line L136 (-84.3689, -81.1004) -> (-84.3689, -88.0286)
  line L137 (-84.3689, -88.0286) -> (-78.3689, -91.4927)
  line L138 (-78.3689, -91.4927) -> (-72.3689, -88.0286)
  line L139 (-72.3689, -88.0286) -> (-72.3689, -81.1004)
  line L140 (-78.3689, -77.6363) -> (-84.3689, -81.1004)
  line L141 (-72.3689, -81.1004) -> (-78.3689, -77.6363)
  line L142 (-70.2022, -81.1004) -> (-70.2022, -88.0286)
  line L143 (-70.2022, -88.0286) -> (-64.2022, -91.4927)
  line L144 (-64.2022, -91.4927) -> (-58.2022, -88.0286)
  line L145 (-58.2022, -88.0286) -> (-58.2022, -81.1004)
  line L146 (-64.2022, -77.6363) -> (-70.2022, -81.1004)
  line L147 (-58.2022, -81.1004) -> (-64.2022, -77.6363)
  line L148 (-56.0355, -81.1004) -> (-56.0355, -88.0286)
  line L149 (-56.0355, -88.0286) -> (-50.0355, -91.4927)
  line L150 (-50.0355, -91.4927) -> (-44.0355, -88.0286)
  line L151 (-44.0355, -88.0286) -> (-44.0355, -81.1004)
  line L152 (-50.0355, -77.6363) -> (-56.0355, -81.1004)
  line L153 (-44.0355, -81.1004) -> (-50.0355, -77.6363)
  line L154 (-41.8689, -81.1004) -> (-41.8689, -88.0286)
  line L155 (-27.7022, -81.1004) -> (-27.7022, -88.0286)
  line L156 (-27.7022, -88.0286) -> (-21.7022, -91.4927)
  line L157 (-21.7022, -91.4927) -> (-15.7022, -88.0286)
  line L158 (-15.7022, -88.0286) -> (-15.7022, -81.1004)
  line L159 (-21.7022, -77.6363) -> (-27.7022, -81.1004)
  line L160 (-15.7022, -81.1004) -> (-21.7022, -77.6363)
  line L161 (-92.5355, -107.4927) -> (-86.5355, -104.0286)
  line L162 (-86.5355, -104.0286) -> (-86.5355, -97.1004)
  line L163 (-86.5355, -97.1004) -> (-92.5355, -93.6363)
  line L164 (-84.3689, -97.1004) -> (-84.3689, -104.0286)
  line L165 (-84.3689, -104.0286) -> (-78.3689, -107.4927)
  line L166 (-78.3689, -107.4927) -> (-72.3689, -104.0286)
  line L167 (-72.3689, -104.0286) -> (-72.3689, -97.1004)
  line L168 (-78.3689, -93.6363) -> (-84.3689, -97.1004)
  line L169 (-72.3689, -97.1004) -> (-78.3689, -93.6363)
  line L170 (-70.2022, -97.1004) -> (-70.2022, -104.0286)
  line L171 (-70.2022, -104.0286) -> (-64.2022, -107.4927)
  line L172 (-64.2022, -107.4927) -> (-58.2022, -104.0286)
  line L173 (-58.2022, -104.0286) -> (-58.2022, -97.1004)
  line L174 (-64.2022, -93.6363) -> (-70.2022, -97.1004)
  line L175 (-58.2022, -97.1004) -> (-64.2022, -93.6363)
  line L176 (-56.0355, -97.1004) -> (-56.0355, -104.0286)
  line L177 (-56.0355, -104.0286) -> (-50.0355, -107.4927)
  line L178 (-50.0355, -107.4927) -> (-44.0355, -104.0286)
  line L179 (-44.0355, -104.0286) -> (-44.0355, -97.1004)
  line L180 (-50.0355, -93.6363) -> (-56.0355, -97.1004)
  line L181 (-44.0355, -97.1004) -> (-50.0355, -93.6363)
  line L182 (-41.8689, -97.1004) -> (-41.8689, -104.0286)
  line L183 (-34.3572, -106.6199) -> (-29.8689, -104.0286)
  line L184 (-29.8689, -104.0286) -> (-29.8689, -97.1004)
  line L185 (-29.8689, -97.1004) -> (-34.3572, -94.509)
  line L186 (-27.7022, -97.1004) -> (-27.7022, -104.0286)
  line L187 (-27.7022, -104.0286) -> (-21.7022, -107.4927)
  line L188 (-21.7022, -107.4927) -> (-15.7022, -104.0286)
  line L189 (-15.7022, -104.0286) -> (-15.7022, -97.1004)
  line L190 (-21.7022, -93.6363) -> (-27.7022, -97.1004)
  line L191 (-15.7022, -97.1004) -> (-21.7022, -93.6363)
  line L192 (-13.5355, -97.1004) -> (-13.5355, -104.0286)
  line L193 (-9.2861, -94.647) -> (-13.5355, -97.1004)
  line L194 (-92.5355, -123.4927) -> (-86.5355, -120.0286)
  line L195 (-86.5355, -120.0286) -> (-86.5355, -113.1004)
  line L196 (-86.5355, -113.1004) -> (-92.5355, -109.6363)
  line L197 (-84.3689, -113.1004) -> (-84.3689, -120.0286)
  line L198 (-84.3689, -120.0286) -> (-78.3689, -123.4927)
  line L199 (-78.3689, -123.4927) -> (-72.3689, -120.0286)
  line L200 (-72.3689, -120.0286) -> (-72.3689, -113.1004)
  line L201 (-78.3689, -109.6363) -> (-84.3689, -113.1004)
  line L202 (-72.3689, -113.1004) -> (-78.3689, -109.6363)
  line L203 (-70.2022, -113.1004) -> (-70.2022, -120.0286)
  line L204 (-70.2022, -120.0286) -> (-64.2022, -123.4927)
  line L205 (-64.2022, -123.4927) -> (-58.2022, -120.0286)
  line L206 (-58.2022, -120.0286) -> (-58.2022, -113.1004)
  line L207 (-64.2022, -109.6363) -> (-70.2022, -113.1004)
  line L208 (-58.2022, -113.1004) -> (-64.2022, -109.6363)
  line L209 (-56.0355, -113.1004) -> (-56.0355, -120.0286)
  line L210 (-56.0355, -120.0286) -> (-50.0355, -123.4927)
  line L211 (-50.0355, -123.4927) -> (-44.0355, -120.0286)
  line L212 (-44.0355, -120.0286) -> (-44.0355, -113.1004)
  line L213 (-50.0355, -109.6363) -> (-56.0355, -113.1004)
  line L214 (-44.0355, -113.1004) -> (-50.0355, -109.6363)
  line L215 (-41.8689, -113.1004) -> (-41.8689, -120.0286)
  line L216 (-29.8689, -120.0286) -> (-29.8689, -113.1004)
  line L217 (-29.8689, -113.1004) -> (-34.3572, -110.509)
  line L218 (-27.7022, -113.1004) -> (-27.7022, -120.0286)
  line L219 (-27.7022, -120.0286) -> (-21.7022, -123.4927)
  line L220 (-21.7022, -123.4927) -> (-15.7022, -120.0286)
  line L221 (-15.7022, -120.0286) -> (-15.7022, -113.1004)
  line L222 (-21.7022, -109.6363) -> (-27.7022, -113.1004)
  line L223 (-15.7022, -113.1004) -> (-21.7022, -109.6363)
  line L224 (-13.5355, -113.1004) -> (-13.5355, -120.0286)
  line L225 (-13.5355, -120.0286) -> (-9.2861, -122.482)
  line L226 (-9.2861, -110.647) -> (-13.5355, -113.1004)
  line L227 (-84.3689, -129.1004) -> (-84.3689, -136.0286)
  line L228 (-72.3689, -136.0286) -> (-72.3689, -129.1004)
  line L229 (-78.3689, -125.6363) -> (-84.3689, -129.1004)
  line L230 (-72.3689, -129.1004) -> (-78.3689, -125.6363)
  line L231 (-70.2022, -129.1004) -> (-70.2022, -136.0286)
  line L232 (-60.6391, -137.4355) -> (-58.2022, -136.0286)
  line L233 (-58.2022, -136.0286) -> (-58.2022, -129.1004)
  line L234 (-64.2022, -125.6363) -> (-70.2022, -129.1004)
  line L235 (-58.2022, -129.1004) -> (-64.2022, -125.6363)
  line L236 (-56.0355, -129.1004) -> (-56.0355, -136.0286)
  line L237 (-46.4725, -137.4355) -> (-44.0355, -136.0286)
  line L238 (-44.0355, -136.0286) -> (-44.0355, -129.1004)
  line L239 (-50.0355, -125.6363) -> (-56.0355, -129.1004)
  line L240 (-44.0355, -129.1004) -> (-50.0355, -125.6363)
  line L241 (-27.7022, -129.1004) -> (-27.7022, -136.0286)
  line L242 (-27.7022, -136.0286) -> (-25.7374, -137.163)
  line L243 (-17.667, -137.163) -> (-15.7022, -136.0286)
  line L244 (-15.7022, -136.0286) -> (-15.7022, -129.1004)
  line L245 (-21.7022, -125.6363) -> (-27.7022, -129.1004)
  line L246 (-15.7022, -129.1004) -> (-21.7022, -125.6363)
  line L247 (-37.5281, -62.5942) -> (-41.8689, -65.1004)
  line L248 (-41.8689, -72.0286) -> (-37.6035, -74.4912)
  line L249 (-84.3689, -136.0286) -> (-81.9319, -137.4355)
  line L250 (-74.8058, -137.4355) -> (-72.3689, -136.0286)
  line L251 (-70.2022, -136.0286) -> (-67.7653, -137.4355)
  line L252 (-56.0355, -136.0286) -> (-53.5986, -137.4355)
  line L253 (-50.5, 0) -> (-50.5, -138.9) construction
  line L254 (-50.5, -139.2245) -> (-50.5, -160) construction
  line L255 (-41.8689, -120.0286) -> (-37.9069, -122.316)
  line L256 (-36, -123.417) -> (-35.8689, -123.4927)
  line L257 (-37.8336, -110.7706) -> (-41.8689, -113.1004)
  line L258 (-41.8689, -104.0286) -> (-37.8058, -106.3744)
  line L259 (-37.7318, -94.7118) -> (-41.8689, -97.1004)
  line L260 (-41.8689, -88.0286) -> (-37.7046, -90.4328)
  line L261 (-37.6299, -78.653) -> (-41.8689, -81.1004)
  line L262 (-84.3689, -52.5645) -> (-72.3689, -52.5645)
  line L263 (-70.2022, -52.5645) -> (-58.2022, -52.5645)
  line L264 (-56.0355, -52.5645) -> (-44.0355, -52.5645)
  line L265 (-92.5355, -75.4927) -> (-92.5355, -61.6363)
  line L266 (-92.5355, -91.4927) -> (-92.5355, -77.6363)
  line L267 (-37.5281, -62.5942) -> (-37.6035, -74.4912)
  line L268 (-37.6299, -78.653) -> (-37.7046, -90.4328)
  line L269 (-37.7318, -94.7118) -> (-37.8058, -106.3744)
  line L270 (-37.8336, -110.7706) -> (-37.9069, -122.316)
  line L271 (-53.5986, -137.4355) -> (-46.4725, -137.4355)
  line L272 (-67.7653, -137.4355) -> (-60.6391, -137.4355)
  line L273 (-81.9319, -137.4355) -> (-74.8058, -137.4355)
  line L274 (-92.5355, -123.4927) -> (-92.5355, -109.6363)
  line L275 (-92.5355, -107.4927) -> (-92.5355, -93.6363)
  line L276 (-35.7372, -77.7123) -> (-35.8689, -77.6363)
  line L277 (-13.5355, -104.0286) -> (-9.2861, -106.482)
  line L278 (-7.8217, -107.3275) -> (-7.5355, -107.4927)
  line L279 (-9.2861, -94.647) -> (-9.2861, -106.482)
  line L280 (-9.2861, -110.647) -> (-9.2861, -122.482)
  line L281 (-34.3572, -106.6199) -> (-34.3572, -94.509)
  line L282 (-17.667, -137.163) -> (-25.7374, -137.163)
  line L283 (-34.3572, -122.6199) -> (-34.3572, -110.509)
  line L284 (-35.8689, -123.4927) -> (-35.8217, -123.4654)
  line L285 (-34.3572, -122.6199) -> (-29.8689, -120.0286)
  line L286 (-35.8217, -125.6635) -> (-35.8689, -125.6363)
  line L287 (-84.3689, -40.0286) -> (-81.8203, -41.5)
  line L288 (-74.9175, -41.5) -> (-72.3689, -40.0286)
  line L289 (-70.2022, -40.0286) -> (-67.6536, -41.5)
  line L290 (-56.0355, -24.0286) -> (-53, -25.7811)
  line L291 (-47.9856, -26.3092) -> (-44.0355, -24.0286)
  line L292 (-60.7508, -41.5) -> (-67.6536, -41.5)
  line L293 (-74.9175, -41.5) -> (-81.8203, -41.5)
  line L294 (-94.007, -26.6431) -> (-94.007, -14.4858)
  line L295 (-53, -15.3478) -> (-53, -25.7811)
  line L296 (-53, -15.3478) -> (-56.0355, -17.1004)
  line L297 (-47.9856, -26.3092) -> (-47.9856, -14.8198)
  line L298 (-32.4175, -41.5) -> (-39.3203, -41.5)
  line L299 (-32.4175, -41.5) -> (-29.8689, -40.0286)
  line L300 (-41.8689, -40.0286) -> (-39.3203, -41.5)
  line L301 (-27.7022, -40.0286) -> (-25.1536, -41.5)
  line L302 (-18.2508, -41.5) -> (-15.7022, -40.0286)
  line L303 (-18.2508, -41.5) -> (-25.1536, -41.5)
  line L304 (-7.5355, -27.4927) -> (-7, -27.1835)
  line L305 (-7, -13.9455) -> (-7, -27.1835)
  line L306 (-89.0676, -2.0505) -> (-89.0676, -5.5)
  line L307 (-89.0676, -5.5) -> (-94, -5.5)
  line L308 (-11, -2.0505) -> (-11, -5)
  line L309 (-11, -5) -> (-11, -6)
  line L310 (-11, -6) -> (-7, -6)
  line L311 (-94.007, -10.6431) -> (-94, -5.5)
  line L312 (-89.0676, -2.0505) -> (-86.5355, -2.0505)
  line L313 (-84.3689, -2.0505) -> (-72.3689, -2.0505)
  line L314 (-70.2022, -2.0505) -> (-58.2022, -2.0505)
  line L315 (-41.8689, -2.0505) -> (-29.8689, -2.0505)
  line L316 (-27.7022, -2.0505) -> (-15.7022, -2.0505)
  line L317 (-13.5355, -2.0505) -> (-11, -2.0505)
  line L318 (-7, -6) -> (-7, -11.1835)
  point P0 (-92.5355, -52.5645)
  constraint midpoint L11 L18.start
  constraint midpoint L13 L18.end
  constraint midpoint L12 L19.start
  constraint midpoint L10 L19.end
  constraint midpoint L15 L20.start
  constraint midpoint L17 L20.end
  constraint midpoint L14 L21.start
  constraint midpoint L16 L21.end
  constraint midpoint L0 L22.start
  constraint midpoint L8 L22.end
  constraint midpoint L9 L23.start
  constraint perpendicular L9 L23
  constraint midpoint L7 L253.start
  constraint midpoint L2 L254.end
  constraint coincident L103.start L262
  constraint coincident L106.end L262
  constraint coincident L110.end L262
  constraint coincident L107.start L262
  constraint coincident L13 L253.end
  constraint collinear L253 L254
  constraint coincident L255.end L267
  constraint coincident L12 L256.start
  constraint collinear L255 L256
  constraint coincident L257.start L267
  constraint coincident L258.end L267
  constraint coincident L259.start L267
  constraint coincident L260.end L267
  constraint coincident L261.start L267
  constraint collinear L262 L263
  constraint collinear L263 L264
  constraint collinear L267 L268
  constraint collinear L268 L269
  constraint collinear L269 L270
  constraint collinear L274 L275
  constraint coincident A8 L276.start
  constraint coincident L16 L278.start
  constraint collinear L277 L278
  constraint collinear L279 L280
  constraint coincident L283.start L284
  constraint coincident L14 L284.end
  constraint collinear L284 L285
  constraint coincident L14 L286.start
  constraint collinear L292 L293
  constraint perpendicular L306 L312
  constraint perpendicular L306 L307
  constraint perpendicular L308 L312
  constraint coincident L27.start L312
  constraint coincident L30.end L312
  constraint collinear L312 L313
  constraint collinear L313 L314
  constraint collinear L315 L316
  constraint collinear L316 L317
extrude "Extrude4" cut sketch "Sketch8" against normal blind 5 contours L31 L32 L33 L34 L314 | L35 L36 L37 L38 L315 | L46 L47 L48 L49 L50 L294 | L57 L58 L59 L60 L61 L62 | L63 L290 L295 L296 | L64 L65 L291 L297 | L66 L67 L68 L69 L70 L71 | L78 L79 L80 L81 L304 L305 | L86 L87 L88 L89 L90 L289 L292 | L91 L92 L93 L94 L298 L299 L300 | L99 L100 L101 L102 L262 | L103 L104 L105 L106 L263 | L107 L108 L109 L110 L264 | L111 L112 L113 L265 | L114 L115 L116 L117 L118 L119 | L120 L121 L122 L123 L124 L125 | L126 L127 L128 L129 L130 L131 | L132 L247 L248 L267 | L133 L134 L135 L266 | L136 L137 L138 L139 L140 L141 | L142 L143 L144 L145 L146 L147 | L148 L149 L150 L151 L152 L153 | L154 L260 L261 L268 | L155 L156 L157 L158 L159 L160 | L161 L162 L163 L275 | L164 L165 L166 L167 L168 L169 | L170 L171 L172 L173 L174 L175 | L176 L177 L178 L179 L180 L181 | L182 L258 L259 L269 | L183 L184 L185 L281 | L186 L187 L188 L189 L190 L191 | L192 L193 L277 L279 | L203 L204 L205 L206 L207 L208 | L209 L210 L211 L212 L213 L214 | L216 L217 L283 L285 | L224 L225 L226 L280 | L231 L232 L233 L234 L235 L251 L272 | L236 L237 L238 L239 L240 L252 L271 bodies 2 in component "chassis"
sketch "Sketch9" plane through (0, 0, 5) normal (0, 0, 1) x (-1, 0, 0)
  line L0 (-95.4377, -42.9681) -> (-95.4377, -1.0386)
  arc A0 (-95.4377, -1.0386) -> (-101, -10) centre (-91, -10) ccw
  line L1 (-101, -10) -> (-101, -150)
  arc A1 (-101, -150) -> (-91, -160) centre (-91, -150) ccw
  line L2 (-91, -160) -> (-10, -160)
  arc A2 (-10, -160) -> (0, -150) centre (-10, -150) ccw
  line L3 (0, -150) -> (0, -10)
  arc A3 (0, -10) -> (-5.5623, -1.0386) centre (-10, -10) ccw
  line L4 (-5.5623, -1.0386) -> (-5.5623, -42.9681)
  line L5 (-5.5623, -42.9681) -> (-49.5623, -42.9681)
  line L6 (-49.5623, -42.9681) -> (-49.5623, 0)
  line L7 (-49.5623, 0) -> (-51.4377, 0)
  line L8 (-51.4377, 0) -> (-51.4377, -42.9681)
  line L9 (-51.4377, -42.9681) -> (-95.4377, -42.9681)
  line L10 (-94, -133.9) -> (-94, -56.1)
  arc A4 (-89, -51.1) -> (-94, -56.1) centre (-89, -56.1) ccw
  line L11 (-89, -51.1) -> (-41, -51.1)
  arc A5 (-36, -56.1) -> (-41, -51.1) centre (-41, -56.1) ccw
  line L12 (-36, -56.1) -> (-36, -133.9)
  arc A6 (-41, -138.9) -> (-36, -133.9) centre (-41, -133.9) ccw
  line L13 (-41, -138.9) -> (-89, -138.9)
  arc A7 (-94, -133.9) -> (-89, -138.9) centre (-89, -133.9) ccw
  line L14 (-35.8217, -133.6274) -> (-35.8217, -78.6274)
  arc A8 (-30.8217, -73.6274) -> (-35.8217, -78.6274) centre (-30.8217, -78.6274) ccw
  line L15 (-30.8217, -73.6274) -> (-12.8217, -73.6274)
  arc A9 (-7.8217, -78.6274) -> (-12.8217, -73.6274) centre (-12.8217, -78.6274) ccw
  line L16 (-7.8217, -78.6274) -> (-7.8217, -133.6274)
  arc A10 (-12.8217, -138.6274) -> (-7.8217, -133.6274) centre (-12.8217, -133.6274) ccw
  line L17 (-12.8217, -138.6274) -> (-30.8217, -138.6274)
  arc A11 (-35.8217, -133.6274) -> (-30.8217, -138.6274) centre (-30.8217, -133.6274) ccw
  line L18 (-50.5, 0) -> (-51.4377, -160) construction
  circle A12 centre (-51.373, -148.9634) radius 1.6
  circle A13 centre (-88.873, -154.9634) radius 1.6
  circle A14 centre (-81.373, -154.9634) radius 1.6
  circle A15 centre (-73.873, -154.9634) radius 1.6
  circle A16 centre (-66.373, -154.9634) radius 1.6
  circle A17 centre (-58.873, -154.9634) radius 1.6
  circle A18 centre (-51.373, -154.9634) radius 1.6
  circle A19 centre (-43.873, -154.9634) radius 1.6
  circle A20 centre (-36.373, -154.9634) radius 1.6
  circle A21 centre (-28.873, -154.9634) radius 1.6
  circle A22 centre (-21.373, -154.9634) radius 1.6
  circle A23 centre (-13.873, -154.9634) radius 1.6
  circle A24 centre (-96.373, -148.9634) radius 1.6
  circle A25 centre (-88.873, -148.9634) radius 1.6
  circle A26 centre (-81.373, -148.9634) radius 1.6
  circle A27 centre (-73.873, -148.9634) radius 1.6
  circle A28 centre (-66.373, -148.9634) radius 1.6
  circle A29 centre (-58.873, -148.9634) radius 1.6
  circle A30 centre (-43.873, -148.9634) radius 1.6
  circle A31 centre (-36.373, -148.9634) radius 1.6
  circle A32 centre (-28.873, -148.9634) radius 1.6
  circle A33 centre (-21.373, -148.9634) radius 1.6
  circle A34 centre (-13.873, -148.9634) radius 1.6
  circle A35 centre (-6.373, -148.9634) radius 1.6
  circle A36 centre (-96.373, -142.9634) radius 1.6
  circle A37 centre (-88.873, -142.9634) radius 1.6
  circle A38 centre (-81.373, -142.9634) radius 1.6
  circle A39 centre (-73.873, -142.9634) radius 1.6
  circle A40 centre (-66.373, -142.9634) radius 1.6
  circle A41 centre (-58.873, -142.9634) radius 1.6
  circle A42 centre (-51.373, -142.9634) radius 1.6
  circle A43 centre (-43.873, -142.9634) radius 1.6
  circle A44 centre (-36.373, -142.9634) radius 1.6
  circle A45 centre (-28.873, -142.9634) radius 1.6
  circle A46 centre (-21.373, -142.9634) radius 1.6
  circle A47 centre (-13.873, -142.9634) radius 1.6
  circle A48 centre (-6.373, -142.9634) radius 1.6
  dimension "d133" = 3.2
  dimension "d136" = 45
  dimension "d137" = 6
  constraint midpoint L7 L18.start
  constraint coincident L2 L18.end
  constraint coincident L18 A12.centre
  measures "d133" diameter of A12
extrude "Extrude6" cut sketch "Sketch9" against normal blind 5 contours A12 | A13 | A14 | A15 | A16 | A17 | A18 | A19 | A20 | A21 | A22 | A23 | A24 | A25 | A26 | A27 | A28 | A29 | A30 | A31 | A32 | A33 | A34 | A35 | A36 | A37 | A38 | A39 | A40 | A41 | A42 | A43 | A44 | A45 | A46 | A47 | A48 bodies 2 in component "chassis"
sketch "Sketch10" plane through (0, 0, 0) normal (-1, 0, 0) x (0, -1, 0)
  line L0 (-150, 5) -> (-150, 0)
  line L1 (-150, 0) -> (-10, 0)
  line L2 (-10, 0) -> (-10, 5)
  line L3 (-10, 5) -> (-150, 5)
  line L4 (-150, 2.5) -> (-10, 2.5) construction
  circle A0 centre (-145, 2.5) radius 1.6
  circle A1 centre (-125.7143, 2.5) radius 1.6
  circle A2 centre (-106.4286, 2.5) radius 1.6
  circle A3 centre (-87.1429, 2.5) radius 1.6
  circle A4 centre (-67.8571, 2.5) radius 1.6
  circle A5 centre (-48.5714, 2.5) radius 1.6
  circle A6 centre (-29.2857, 2.5) radius 1.6
  dimension "d140" = 3.2
  constraint midpoint L0 L4.start
  constraint midpoint L2 L4.end
  constraint coincident L4 A0.centre
  measures "d140" diameter of A0
extrude "Extrude7" cut sketch "Sketch10" against normal blind 5 contours A0 | A1 | A2 | A3 | A4 | A5 | A6 bodies 2 in component "chassis"
ref_plane "WorkPlane2" through (50.5, 80, 2.5) normal (-1, 0, 0) x (0, -1, 0)
mirror "Mirror1'" about plane through (50.5, 80, 2.5) normal (-1, 0, 0) of "Extrude7" in component "chassis"